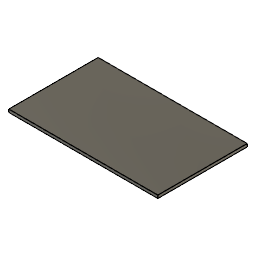
Enclosure Top (Autodesk Fusion 360 design; units mm, degrees)
part number: 2026-03-16-08-46-47-074
Autodesk Fusion 360 part; units mm, degrees
sketch "Sketch1" plane through (0, 0, 0) normal (0, 0, 1) x (1, 0, 0)
  line L0 (-61.008, 52.2356) -> (188.992, 52.2356)
  line L1 (188.992, 52.2356) -> (188.992, -97.7644)
  line L2 (188.992, -97.7644) -> (-61.008, -97.7644)
  line L3 (-61.008, -97.7644) -> (-61.008, 52.2356)
  dimension "d1" = 250
  dimension "d2" = 150
  constraint horizontal L0
  constraint vertical L1
  constraint horizontal L2
  constraint vertical L3
  measures "d1" distance of L0.start L0.end
  measures "d2" distance of L0.start L2.end
extrude "Extrude1" add sketch "Sketch1" along normal blind 5
